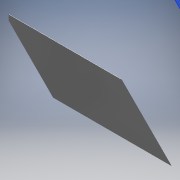
# Autodesk Inventor part: Side Plates
Saved by Autodesk Inventor 2019.4 (Build 234330000, 330)
## iProperties
Created: 2020-01-19
Part Number: Side Plates
Material: Aluminum 6061
Document SubType Name: Modeling
Designer: Mark
Mass: 230.31 g
Surface Area: 1720.09 cm^2
Volume: 85.3 cm^3
Density: 2.7 g/cm^3
Appearance: Aluminum - Flat
Author: Mark
Autodesk Inventor part; units mm, degrees
ref_plane "YZ Plane" through (0, 0, 0) normal (1, 0, 0) x (0, 1, 0)
ref_plane "XZ Plane" through (0, 0, 0) normal (0, 1, 0) x (-1, 0, 0)
ref_plane "XY Plane" through (0, 0, 0) normal (0, 0, 1) x (1, 0, 0)
sketch "Sketch1" plane through (0, 0, 0) normal (0, 0, 1) x (1, 0, 0)
  line L0 (-260, 0) -> (0, 0)
  line L1 (0, 0) -> (0, 190)
  line L2 (0, 190) -> (-430, 190)
  line L3 (-430, 190) -> (-430, 170)
  line L4 (0, -25.9599) -> (0, 190) construction
  line L5 (0, 0) -> (-430, 190) construction
  line L6 (0, 190) -> (190, 0)
  line L7 (190, 0) -> (0, 0)
  line L8 (-430, 190) -> (-430, 170)
  line L9 (-430, 190) -> (-410, 190) construction
  line L10 (-430, 170) -> (-260, 0)
  dimension "d0" = 430
  dimension "d1" = 190
  dimension "d2" = 45
  dimension "d3" = 20
  dimension "d4" = 90
  dimension "d5" = 135
  constraints: 23 end point, 3 perpendicular, 2 horizontal, 2 parallel, 1 collinear, 1 point on line
  measures "d0" distance of L2.end L1.end
  measures "d1" distance of L0.end L1.end
  measures "d2" angle of L1 L6
  measures "d3" distance of L3.end L2.end
  measures "d4" angle of L8 L9
  measures "d5" angle of L0 L10
extrude "Extrusion1" add sketch "Sketch1" along normal blind 1
sketch "Sketch2" plane through (0, 0, 1) normal (0, 0, 1) x (1, 0, 0)
  point P0 (0, 0)
body "Solid1"
